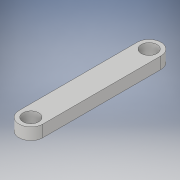
# Autodesk Inventor part: 000.704 - Тяга
Saved by Autodesk Inventor 2019 (Build 230136000, 136)
## iProperties
Created: 2020-02-29
Part Number: 000.704 - Тяга
Material: Типовые
Document SubType Name: Modeling
Designer: Петров Иван
Density: 1 g/cm^3
Appearance: По умолчанию
Author: Петров Иван
Autodesk Inventor part; units mm, degrees
ref_plane "YZ Plane" through (0, 0, 0) normal (1, 0, 0) x (0, 1, 0)
ref_plane "XZ Plane" through (0, 0, 0) normal (0, 1, 0) x (-1, 0, 0)
ref_plane "XY Plane" through (0, 0, 0) normal (0, 0, 1) x (1, 0, 0)
sketch "Эскиз1" plane through (0, 0, 0) normal (0, 1, 0) x (-1, 0, 0)
  line L0 (0, 0) -> (0, -15) construction
  line L1 (-3, 0) -> (-3, -15)
  line L2 (3, -15) -> (3, 0)
  arc A0 (3, 0) -> (-3, 0) centre (0, 0) ccw
  arc A1 (-3, -15) -> (3, -15) centre (0, -15) ccw
  circle A2 centre (0, -15) radius 2
  point P0 (0, -7.5)
  dimension "d0" = 15
  dimension "d1" = 6
  dimension "d2" = 4
  constraints: 8 end point, 4 point on circle, 4 tangent, 3 centre point, 1 coincident, 1 midpoint, 1 parallel, 1 vertical
  measures "d0" distance of L0.start L0.end
  measures "d1" diameter of A1
  measures "d2" diameter of A2
extrude "Выдавливание1" add sketch "Эскиз1" along normal blind 3
pattern_circular "Круговой массив1" count 2 over 360 about axis through (0, 0, 0) along (0, 1, 0) of "Выдавливание1"
